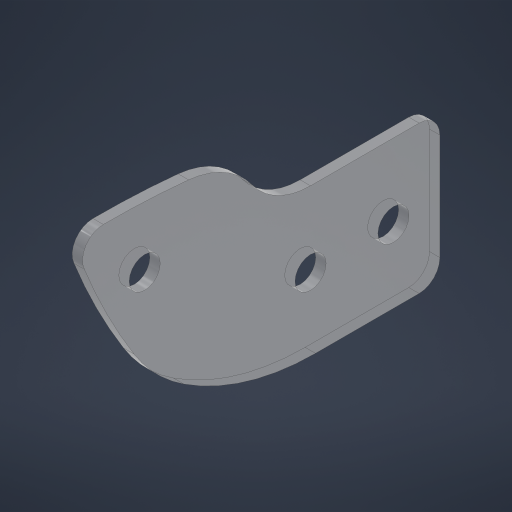
# Autodesk Inventor part: sled
Saved by Autodesk Inventor 2024 (Build 280153000, 153)
## iProperties
Created: 2024-01-29
Part Number: sled
Material: Generic
Document SubType Name: Modeling
Designer: macbook
Density: 1 g/cm^3
Appearance: Polycarbonate - Clear(1)
Author: macbook
Autodesk Inventor part; units mm, degrees
ref_plane "YZ Plane" through (0, 0, 0) normal (1, 0, 0) x (0, 1, 0)
ref_plane "XZ Plane" through (0, 0, 0) normal (0, 1, 0) x (-1, 0, 0)
ref_plane "XY Plane" through (0, 0, 0) normal (0, 0, 1) x (1, 0, 0)
sketch "Sketch2" plane through (0, 0, 0) normal (1, 0, 0) x (0, 1, 0)
  line L0 (-10.5343, 1.8326) -> (14.8657, 1.8326) construction
  line L1 (-10.5343, 1.8326) -> (-23.2343, 1.8326)
  line L2 (14.8657, 1.8326) -> (14.8657, 33.5826)
  line L3 (14.8657, 33.5826) -> (21.2157, 33.5826)
  arc A0 (24.3907, 33.5692) -> (18.0407, 33.5826) centre (21.2157, 33.5826) ccw
  line L4 (-10.5343, 1.8326) -> (-10.5343, 27.2326)
  line L5 (21.2157, 33.5826) -> (19.8929, 33.5826)
  arc A1 (18.4214, -5.6206) -> (24.3907, 33.5692) centre (-103.5619, 33.0092) ccw
  line L6 (21.1383, 36.7567) -> (20.6141, 36.7567)
  arc A2 (20.207, 36.5931) -> (4.8725, 28.8882) centre (54.3249, -50.4207) ccw
  arc A3 (-6.7994, 20.2847) -> (-12.9991, 12.2415) centre (9.812, 1.0696) ccw
  line L7 (-10.5343, 1.8326) -> (-10.5395, -10.8674)
  line L8 (-10.5395, -10.8674) -> (2.1605, -10.8727)
  arc A4 (14.8657, -15.4374) -> (16.4404, -11.3937) centre (-103.5619, 33.0092) ccw
  arc A5 (18.4214, -5.6206) -> (14.8657, -28.6257) centre (91.0657, -28.6257) ccw
  line L9 (14.8657, 1.8326) -> (14.8657, 27.2326)
  line L10 (14.8657, 33.5826) -> (-10.5343, 33.5826)
  line L11 (2.1605, -10.8727) -> (2.1605, -17.9797)
  line L12 (2.1605, -17.9797) -> (10.4725, -17.9797)
  line L13 (2.1605, -17.9797) -> (-5.7795, -17.9797)
  line L14 (-8.9545, -14.8047) -> (-8.9545, 1.0703)
  line L15 (13.6475, -14.8047) -> (13.6475, 1.8326)
  arc A6 (-2.9466, 21.2359) -> (-8.9545, 1.0703) centre (27.8921, 1.0703) ccw
  arc A7 (4.8725, 28.8882) -> (-2.9466, 21.2359) centre (18.3119, 7.3349) ccw
  arc A8 (16.4403, 9.623) -> (23.7808, 20.5184) centre (10.0212, 21.8681) ccw
  arc A9 (18.1559, 10.6889) -> (13.6475, 1.8326) centre (24.6004, 1.8326) ccw
  arc A10 (10.4725, -17.9797) -> (13.6475, -14.8047) centre (10.4725, -14.8047) ccw
  arc A11 (-8.9545, -14.8047) -> (-5.7795, -17.9797) centre (-5.7795, -14.8047) ccw
  line L16 (2.1605, -10.8727) -> (2.1605, 1.8273)
  point P0 (0, 0)
  point P1 (13.6475, -17.9797)
  point P2 (-8.9545, -17.9797)
  point P3 (-8.9545, -10.868)
  point P4 (19.8992, 36.4718)
  dimension "d0" = 25.4
  dimension "d1" = 12.7
  dimension "d2" = 6.35
  dimension "d3" = 6.35
  dimension "d4" = 31.75
  dimension "d5" = 25.4
  dimension "d7" = 25.4
  dimension "d8" = 12.7
  dimension "d12" = 25.4
  dimension "d17" = 19.05
  dimension "d18" = 25.4
  dimension "d21" = 3.175
  dimension "d29" = 12.7
  constraints: 34 end point, 31 point on circle, 12 centre point, 12 tangent, 7 point on line, 5 horizontal, 5 vertical, 4 coincident, 3 perpendicular, 1 equal radius, 1 midpoint
  measures "d0" distance of L0.start L9.start
  measures "d1" distance of L0.start L1.end
  measures "d2" distance of L2.end L3.end
  measures "d3" diameter of A0
  measures "d4" distance of L9.start L2.end
  measures "d5" distance of L0.start L4.end
  measures "d7" radius of A3
  measures "d8" distance of L0.start L7.end
  measures "d12" distance of L2.end L10.end
  measures "d17" distance of point (-8.955, -17.98) L14.end
  measures "d18" radius of A7
  measures "d21" radius of A10
  measures "d29" distance of L11.start L16.end
extrude "Extrusion1" add sketch "Sketch2" along normal blind 1.5875
hole "Hole1" at (0, 14.8657, 27.2326) at (0, 2.1605, -10.8727) at (0, 2.1605, 1.8273) direction (1, 0, 0) diameter 4.7625 end through all
body "Solid1"
